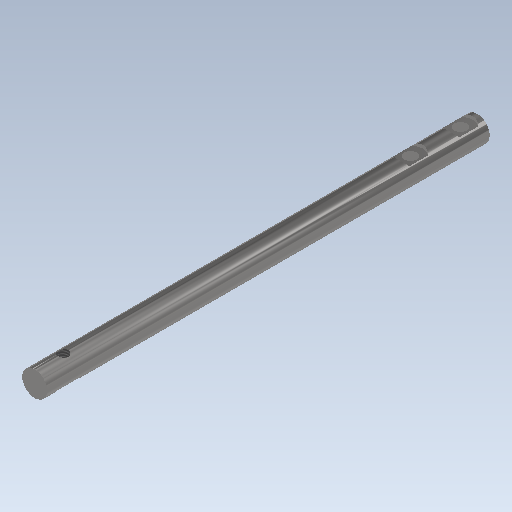
# Autodesk Inventor part: PWTR-0031
Saved by Autodesk Inventor 2021.1 (Build 251245010, 245A)
## iProperties
Shininess: 64.0
Length Units: 11269
Angle Units: 11279
Time Units: 11290
Mass Units: 11284
Length Display Precision: 3
Angle Display Precision: 2
Compacted: True
Part Number: PWTR-0031
Document SubType Name: Modeling
Created: 2003-02-05
Designer: B. BOGAN
Description: Trowel Arm
Material: Stainless Steel, 303
Density: 7.75 g/cm^3
Appearance: Steel - Polished
Mass: 258.875 g
Surface Area: 116.731 cm^2
Volume: 33.4032 cm^3
Vendor: Non-Design Specific
Density: 0.0
Volumn: 0.0
Area: 0.0
PropertySet Name: Model Information
Control State: 0
Master: False
Checked Out: False
Title: TROWEL ARM
Author: B. BOGAN
Revision Number: B
Autodesk Inventor part; units mm, degrees
ref_plane "YZ Plane" through (0, 0, 0) normal (1, 0, 0) x (0, 1, 0)
sketch "Sketch1" plane through (0, 0, 0) normal (0, 0, 1) x (1, 0, 0)
  circle A0 centre (0, 0) radius 6.35
  dimension "d0" = 12.7
  constraints: 1 centre point
  measures "d0" diameter of A0
extrude "Extrusion1" add sketch "Sketch1" along normal blind 225
ref_plane "Work Plane2" through (0, 0, 218.4976) normal (0, 0, 1) x (1, 0, 0)
sketch "Sketch2" plane through (0, 0, 218.4976) normal (0, 0, 1) x (1, 0, 0)
  circle A0 centre (0, 0) radius 6.35
  line L0 (-5.4993, -3.175) -> (5.4993, -3.175)
  dimension "d3" = 9.525
  constraints: 2 end point, 2 point on circle, 1 centre point, 1 horizontal
extrude "Extrusion3" cut sketch "Sketch2" against normal blind 12.7762 contours L0 A0 picked at (-1.5396, -3.5692)
sketch "Sketch3" plane through (-5.4993, -3.175, 218.4976) normal (0, -1, 0) x (1, 0, 0)
  line L0 (0, 0) -> (10.9985, 0)
  line L1 (10.9985, -12.7762) -> (0, -12.7762) projected
  line L2 (10.9985, 0) -> (10.9985, -12.7762) projected
  line L3 (10.9985, 0) -> (0, 0) projected
  line L4 (0, -12.7762) -> (0, 0) projected
  point P0 (5.4993, -7.9756)
  dimension "d6" = 7.9756
  constraints: 2 end point
  measures "d6" distance from line of point (5.499, -7.976) L0
hole "Hole1" at (0, -3.175, 210.522) direction (0, 1, 0) diameter 5.2578 end through all thread size "1/4-20 UNC" class "2B" standard "ANSI Unified Screw Threads"
ref_plane "Work Plane1" through (0, 6.35, 0) normal (0, 1, 0) x (-1, 0, 0)
sketch "Sketch4" plane through (0, 6.35, 0) normal (0, 1, 0) x (-1, 0, 0)
  line L0 (-6.35, 0) -> (6.35, 0) projected
  point P0 (0, 8.5)
  point P1 (0, 33.9)
  point P2 (0, 210.522)
  dimension "d14" = 25.4
  dimension "d28" = 8.5
  constraints: 1 vertical alignment
  measures "d14" distance of point (0, 33.9) point (0, 8.5)
  measures "d28" distance from line of L0 point (0, 8.5)
hole "Hole2" at (0, 6.35, 8.5) at (0, 6.35, 33.9) direction (0, -1, 0) diameter 6.35 end through all counterbore diameter 12.7 counterbore depth 1.5875
body "Solid1"
